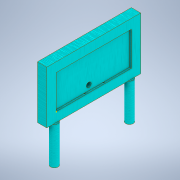
# Autodesk Inventor part: upper part edited
Saved by Autodesk Inventor 2021.3 (Build 253353000, 353)
## iProperties
Created: 2021-07-03
Part Number: upper part edited
Material: Polyethylene, High Density
Document SubType Name: Modeling
Designer: ASUS
Density: 0.952 g/cm^3
Appearance: Smooth - Off-White
Author: ASUS
Autodesk Inventor part; units mm, degrees
ref_plane "YZ Plane" through (0, 0, 0) normal (1, 0, 0) x (0, 1, 0)
ref_plane "XZ Plane" through (0, 0, 0) normal (0, 1, 0) x (-1, 0, 0)
ref_plane "XY Plane" through (0, 0, 0) normal (0, 0, 1) x (1, 0, 0)
sketch "Sketch1" plane through (0, 0, 0) normal (1, 0, 0) x (0, 1, 0)
  line L0 (46, 10) -> (-10, 10)
  line L1 (46, -90) -> (-10, -90)
  line L2 (46, 10) -> (46, -90)
  line L3 (-10, 10) -> (-10, -90)
  point P0 (0, 0)
  dimension "d4" = 100
  constraints: 8 end point, 2 horizontal, 1 parallel, 1 vertical
  measures "d4" distance of L1.end L0.end
extrude "Extrusion1" add sketch "Sketch1" along normal blind 10
sketch "Sketch2" plane through (10, 0, 0) normal (1, 0, 0) x (0, 0, -1)
  line L0 (0, 36) -> (80, 36)
  line L1 (80, 36) -> (80, 0)
  line L2 (80, 0) -> (0, 0)
  line L3 (0, 0) -> (0, 36)
  line L4 (90, 46) -> (-10, 46) projected
  line L5 (-10, -10) -> (90, -10) projected
  line L6 (-10, 46) -> (-10, -10) projected
  line L7 (90, -10) -> (90, 46) projected
  point P0 (0, 0)
  dimension "d9" = 80
  dimension "d10" = 36
  dimension "d11" = 10
  dimension "d12" = 10
  dimension "d13" = 10
  dimension "d14" = 10
  constraints: 8 end point, 2 parallel, 1 horizontal, 1 perpendicular
  measures "d9" distance of L1.end L2.end
  measures "d10" distance of L1.end L0.end
  measures "d11" distance between parallel lines of L0 L4
  measures "d12" distance between parallel lines of L5 L2
  measures "d13" distance between parallel lines of L6 L3
  measures "d14" distance between parallel lines of L7 L1
extrude "Extrusion2" cut sketch "Sketch2" against normal blind 2 contours L0 L1 L2 L3
sketch "Sketch3" plane through (10, 0, 0) normal (0, 1, 0) x (1, 0, 0)
  circle A0 centre (-2.8864, 52.3034) radius 1.5
  circle A1 centre (-2.8864, 32.3034) radius 1.5
  line L0 (0, 80) -> (-2, 80) projected
  line L1 (0, 0) -> (-2, 0) projected
  point P0 (-10, 0)
  dimension "d17" = 3
  dimension "d18" = 3
  dimension "d19" = 20
  dimension "d20" = 27.6966
  dimension "d21" = 32.3034
  constraints: 2 centre point
  measures "d17" diameter of A0
  measures "d18" diameter of A1
  measures "d19" distance of A0.centre A1.centre
  measures "d20" distance from line of L0 A0.centre
  measures "d21" distance from line of L1 A1.centre
extrude "Extrusion3" cut sketch "Sketch3" against normal through all
sketch "Sketch4" plane through (8, 0, 0) normal (1, 0, 0) x (0, 0, -1)
  circle A0 centre (36.6715, 5.3743) radius 2.5605
  point P0 (0, 0)
  constraints: 1 centre point
extrude "Extrusion4" cut sketch "Sketch4" against normal through all
sketch "Sketch5" plane through (0, -10, -90) normal (0, -1, 0) x (1, 0, 0)
  line L0 (8, 10) -> (8, 90) projected
  circle A0 centre (8, 90) radius 4
  line L1 (10, 10) -> (8, 10) projected
  circle A1 centre (8, 10) radius 4
  point P0 (0, 90)
  dimension "d26" = 8
  dimension "d27" = 8
  constraints: 2 centre point, 1 coincident
  measures "d26" diameter of A0
  measures "d27" diameter of A1
extrude "Extrusion5" add sketch "Sketch5" along normal blind 40
sketch "Sketch6" plane through (0, -10, -90) normal (0, -1, 0) x (1, 0, 0)
  point P0 (0, 90)
sketch "Sketch8" plane through (0, -10, -90) normal (0, -1, 0) x (1, 0, 0)
  point P0 (0, 90)
sketch "Sketch9" plane through (10, 0, 0) normal (1, 0, 0) x (0, 0, -1)
  point P0 (0, 0)
sketch "Sketch10" plane through (0, 0, 0) normal (-1, 0, 0) x (0, 0, 1)
  line L0 (-78.8319, 36.3964) -> (1.1681, 36.3964)
  line L1 (1.1681, 36.3964) -> (1.1681, 0.3964)
  line L2 (1.1681, 0.3964) -> (-78.8319, 0.3964)
  line L3 (-78.8319, 0.3964) -> (-78.8319, 36.3964)
  point P0 (0, 0)
  dimension "d34" = 80
  dimension "d35" = 36
  constraints: 8 end point, 2 parallel, 1 horizontal, 1 perpendicular
  measures "d34" distance of L1.end L2.end
  measures "d35" distance of L0.end L1.end
extrude "Extrusion7" cut sketch "Sketch10" against normal blind 2
body "Solid1"
